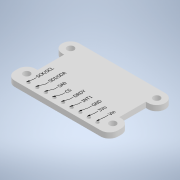
# Autodesk Inventor part: L3GD20H footprint
Saved by Autodesk Inventor 2020 (Build 240168000, 168)
## iProperties
Created: 2020-09-26
Part Number: L3GD20H footprint
Material: Generic
Document SubType Name: Modeling
Designer: mulve
Density: 1 g/cm^3
Appearance: Default
Author: mulve
Autodesk Inventor part; units mm, degrees
ref_plane "YZ Plane" through (0, 0, 0) normal (1, 0, 0) x (0, 1, 0)
ref_plane "XZ Plane" through (0, 0, 0) normal (0, 1, 0) x (-1, 0, 0)
ref_plane "XY Plane" through (0, 0, 0) normal (0, 0, 1) x (1, 0, 0)
sketch "Sketch1" plane through (0, 0, 0) normal (0, 1, 0) x (-1, 0, 0)
  line L0 (-2.54, 0) -> (-27.94, 0)
  line L1 (-30.48, -16.51) -> (-30.48, -16.51)
  line L2 (-27.94, -19.05) -> (-2.54, -19.05)
  line L3 (0, -16.51) -> (0, -16.51)
  circle A0 centre (-2.54, -16.51) radius 1.016
  circle A1 centre (-27.94, -16.51) radius 1.016
  circle A2 centre (-2.54, -3.556) radius 1.016
  circle A3 centre (-27.94, -3.556) radius 1.016
  line L4 (-3.175, -19.05) -> (-27.305, -19.05)
  line L5 (-27.305, -19.05) -> (-27.305, 0)
  line L6 (-27.305, 0) -> (-3.175, 0)
  line L7 (-3.175, 0) -> (-3.175, -19.05)
  line L8 (-2.54, -13.97) -> (-27.94, -13.97)
  line L9 (-30.48, -13.97) -> (-30.48, -6.096)
  line L10 (-27.94, -6.096) -> (-2.54, -6.096)
  line L11 (0, -6.096) -> (0, -13.97)
  arc A4 (-2.54, -19.05) -> (0, -16.51) centre (-2.54, -16.51) ccw
  arc A5 (-30.48, -16.51) -> (-27.94, -19.05) centre (-27.94, -16.51) ccw
  arc A6 (0, -16.51) -> (-2.54, -13.97) centre (-2.54, -16.51) ccw
  arc A7 (-27.94, -13.97) -> (-30.48, -16.51) centre (-27.94, -16.51) ccw
  line L12 (0, -3.556) -> (0, -2.54)
  line L13 (-30.48, -3.556) -> (-30.48, -2.54)
  arc A8 (-30.48, -3.556) -> (-27.94, -6.096) centre (-27.94, -3.556) ccw
  arc A9 (-27.94, 0) -> (-30.48, -2.54) centre (-27.94, -2.54) ccw
  arc A10 (0, -2.54) -> (-2.54, 0) centre (-2.54, -2.54) ccw
  arc A11 (-2.54, -6.096) -> (0, -3.556) centre (-2.54, -3.556) ccw
  line L14 (-0.2121, -1.524) -> (-30.2679, -1.524) construction
  circle A12 centre (-5.08, -1.524) radius 0.508
  circle A13 centre (-7.62, -1.524) radius 0.508
  circle A14 centre (-10.16, -1.524) radius 0.508
  circle A15 centre (-12.7, -1.524) radius 0.508
  circle A16 centre (-15.24, -1.524) radius 0.508
  circle A17 centre (-17.78, -1.524) radius 0.508
  circle A18 centre (-20.32, -1.524) radius 0.508
  circle A19 centre (-22.86, -1.524) radius 0.508
  circle A20 centre (-25.4, -1.524) radius 0.508
  point P0 (0, 0)
  point P1 (-30.48, -19.05)
  point P2 (-30.48, 0)
  point P3 (0, -19.05)
  point P4 (-3.175, -13.97)
  point P5 (-3.175, -6.096)
  point P6 (-27.305, -6.096)
  point P7 (-27.305, -13.97)
  dimension "d0" = 30.48
  dimension "d1" = 19.05
  dimension "d2" = 3.556
  dimension "d3" = 3.556
  dimension "d4" = 2.54
  dimension "d5" = 2.54
  dimension "d6" = 2.54
  dimension "d7" = 2.54
  dimension "d8" = 12.954
  dimension "d9" = 12.954
  dimension "d10" = 2.032
  dimension "d11" = 24.13
  dimension "d12" = 3.175
  dimension "d13" = 3.175
  dimension "d14" = 2.54
  dimension "d15" = 2.54
  dimension "d16" = 2.54
  dimension "d17" = 2.54
  dimension "d18" = 1.524
  dimension "d19" = 5.08
  dimension "d22" = 2.54
  dimension "d27" = 5.08
  dimension "d28" = 1.016
  dimension "d31" = 2.54
  constraints: 30 end point, 21 centre point, 19 point on line, 18 point on circle, 16 tangent, 9 equal radius, 7 parallel, 5 coincident, 5 horizontal, 5 perpendicular, 2 collinear, 24 other
  measures "d0" distance of point (-30.48, -19.05) point (0, -19.05)
  measures "d1" distance of point (-30.48, 0) point (-30.48, -19.05)
  measures "d2" distance from line of L0 point (-27.94, -3.556)
  measures "d3" distance from line of L0 point (-2.54, -3.556)
  measures "d4" distance from line of L3 point (-2.54, -3.556)
  measures "d5" distance from line of L1 point (-27.94, -3.556)
  measures "d6" distance from line of L1 point (-27.94, -16.51)
  measures "d7" distance from line of L3 point (-2.54, -16.51)
  measures "d8" distance of point (-2.54, -3.556) point (-2.54, -16.51)
  measures "d9" distance of point (-27.94, -3.556) point (-27.94, -16.51)
  measures "d10" diameter of A0
  measures "d11" distance of L4.start L4.end
  measures "d12" distance between parallel lines of L3 L7
  measures "d13" distance between parallel lines of L1 L5
  measures "d14" distance from line of L8 A0.centre
  measures "d15" distance from line of L10 A2.centre
  measures "d16" radius of A4
  measures "d17" radius of A8
  measures "d18" distance between parallel lines of L0 L14
  measures "d19" distance from line of L12 point (-5.08, -1.524)
  measures "d22" distance of point (-5.08, -1.524) point (-7.62, -1.524)
  measures "d27" distance from line of L13 point (-25.4, -1.524)
  measures "d28" diameter of A12
  measures "d31" distance of A12.centre A13.centre
extrude "Extrusion1" add sketch "Sketch1" along normal blind 1.6 contours A10 L12 A11 L10 L7 A2 L0 | L7 A2 L10 L5 A3 L0 | L5 A3 L10 A8 L13 A9 L0 | L7 L8 L5 L10 | L8 A6 A4 L2 L7 A0 | L7 A0 L2 L5 A1 L8 | L5 A1 L2 A5 A7 L8
equation "\"d3\" = d2"
equation "\"d9\" = d8"
equation "\"d12\" = d13"
equation "\"d19\" = d27"
body "Solid1"
